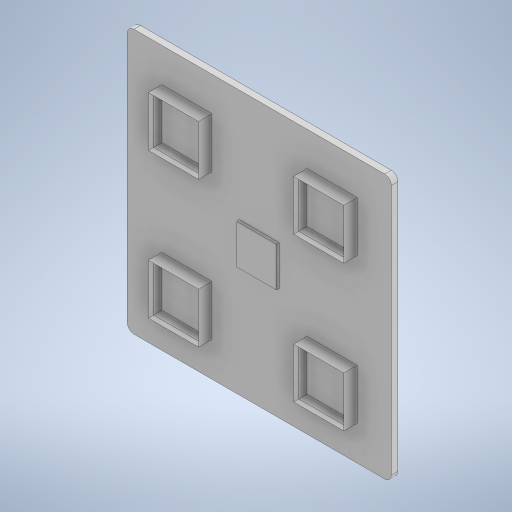
# Autodesk Inventor part: testovaci_podlozka
Saved by Autodesk Inventor 2023 (Build 270158000, 158)
## iProperties
Created: 2025-03-28
Part Number: testovaci_podlozka
Material: Všeobecné
Document SubType Name: Modeling
Designer: lisnik
Density: 1 g/cm^3
Appearance: Výchozí
Author: lisnik
Autodesk Inventor part; units mm, degrees
ref_plane "YZ Plane" through (0, 0, 0) normal (1, 0, 0) x (0, 1, 0)
ref_plane "XZ Plane" through (0, 0, 0) normal (0, 1, 0) x (-1, 0, 0)
ref_plane "XY Plane" through (0, 0, 0) normal (0, 0, 1) x (1, 0, 0)
sketch "Náčrt1" plane through (0, 0, 0) normal (0, 0, 1) x (1, 0, 0)
  line L0 (-140, 0) -> (140, 0) projected
  line L1 (0, -140) -> (0, 140) projected
  line L2 (-100, 100) -> (100, 100)
  line L3 (100, 100) -> (100, -100)
  line L4 (100, -100) -> (-100, -100)
  line L5 (-100, -100) -> (-100, 100)
  point P0 (0, 0)
  point P1 (0, 100)
  point P2 (100, 0)
  dimension "d0" = 200
  dimension "d1" = 200
  constraints: 8 end point, 2 midpoint, 2 parallel, 2 point on line, 1 horizontal, 1 perpendicular
  measures "d0" distance of L3.end L4.end
  measures "d1" distance of L2.end L3.end
extrude "Vysunutí1" add sketch "Náčrt1" along normal blind 5
fillet "Zaoblení1" radius 5 4 edges at (100, 100, 2.5) (-100, 100, 2.5) (-100, -100, 2.5) (100, -100, 2.5)
sketch "Náčrt2" plane through (0, 0, 5) normal (0, 0, 1) x (1, 0, 0)
  line L0 (-100, 95) -> (-100, -95) projected
  line L1 (-95, -100) -> (95, -100) projected
  arc A0 (95, -100) -> (100, -95) centre (95, -95) ccw projected
  line L2 (100, -95) -> (100, 95) projected
  arc A1 (100, 95) -> (95, 100) centre (95, 95) ccw projected
  line L3 (95, 100) -> (-95, 100) projected
  arc A2 (-95, 100) -> (-100, 95) centre (-95, 95) ccw projected
  line L4 (-100, 95) -> (-100, -95) projected
  arc A3 (-100, -95) -> (-95, -100) centre (-95, -95) ccw projected
  line L5 (-95, -100) -> (95, -100) projected
  line L6 (-141.4497, 0) -> (141.4497, 0) projected
  line L7 (0, -141.4497) -> (0, 141.4497) projected
  line L8 (-15, -15) -> (15, -15)
  line L9 (15, -15) -> (15, 15)
  line L10 (15, 15) -> (-15, 15)
  line L11 (-15, 15) -> (-15, -15)
  line L12 (-72, -72) -> (-38, -72)
  line L13 (-38, -72) -> (-38, -38)
  line L14 (-38, -38) -> (-72, -38)
  line L15 (-72, -38) -> (-72, -72)
  line L16 (-72, 38) -> (-38, 38)
  line L17 (-72, 72) -> (-72, 38)
  line L18 (-38, 72) -> (-72, 72)
  line L19 (-38, 38) -> (-38, 72)
  line L20 (38, -72) -> (72, -72)
  line L21 (38, -38) -> (38, -72)
  line L22 (72, -38) -> (38, -38)
  line L23 (72, -72) -> (72, -38)
  line L24 (38, 38) -> (72, 38)
  line L25 (38, 72) -> (38, 38)
  line L26 (72, 72) -> (38, 72)
  line L27 (72, 38) -> (72, 72)
  point P0 (0, 0)
  point P1 (-15, 0)
  point P2 (0, 15)
  dimension "d5" = 30
  dimension "d6" = 30
  dimension "d8" = 34
  dimension "d9" = 34
  dimension "d10" = 28
  dimension "d11" = 28
  dimension "d14" = 110
  dimension "d17" = 110
  constraints: 40 end point, 4 parallel, 3 horizontal, 2 midpoint, 2 perpendicular, 2 point on line, 1 vertical, 24 other
  measures "d5" distance of L8.end L9.end
  measures "d6" distance of L9.end L10.end
  measures "d8" distance of L13.start L13.end
  measures "d9" distance of L13.end L14.end
  measures "d10" distance between parallel lines of L5 L12
  measures "d11" distance between parallel lines of L0 L15
  measures "d14" distance of L15.end L16.start
  measures "d17" distance of L15.end L20.start
extrude "Vysunutí2" add sketch "Náčrt2" along normal blind 2 contours L11 L10 L7 L6 | L6 L7 L8 L11 | L7 L10 L9 L6 | L6 L9 L8 L7 | L15 L14 L13 L12 | L17 L18 L19 L16 | L21 L22 L23 L20 | L25 L26 L27 L24
sketch "Náčrt4" plane through (0, 0, 5) normal (0, 0, 1) x (1, 0, 0)
  line L0 (-38, 38) -> (-72, 38) projected
  line L1 (-72, 38) -> (-72, 72) projected
  line L2 (-72, 72) -> (-38, 72) projected
  line L3 (-38, 72) -> (-38, 38) projected
  line L4 (72, 38) -> (38, 38) projected
  line L5 (38, 38) -> (38, 72) projected
  line L6 (38, 72) -> (72, 72) projected
  line L7 (72, 72) -> (72, 38) projected
  line L8 (-15, 15) -> (15, 15) projected
  line L9 (15, 15) -> (15, -15) projected
  line L10 (15, -15) -> (-15, -15) projected
  line L11 (-15, -15) -> (-15, 15) projected
  line L12 (72, -72) -> (38, -72) projected
  line L13 (38, -72) -> (38, -38) projected
  line L14 (38, -38) -> (72, -38) projected
  line L15 (72, -38) -> (72, -72) projected
  line L16 (-38, -38) -> (-38, -72) projected
  line L17 (-38, -72) -> (-72, -72) projected
  line L18 (-72, -72) -> (-72, -38) projected
  line L19 (-72, -38) -> (-38, -38) projected
  arc A0 (95, -100) -> (100, -95) centre (95, -95) ccw projected
  line L20 (100, -95) -> (100, 95) projected
  arc A1 (100, 95) -> (95, 100) centre (95, 95) ccw projected
  line L21 (95, 100) -> (-95, 100) projected
  arc A2 (-95, 100) -> (-100, 95) centre (-95, 95) ccw projected
  line L22 (-100, 95) -> (-100, -95) projected
  arc A3 (-100, -95) -> (-95, -100) centre (-95, -95) ccw projected
  line L23 (-95, -100) -> (95, -100) projected
  line L24 (-38, -38) -> (-72, -38) projected
  line L25 (-72, -38) -> (-72, -72) projected
  line L26 (-72, -72) -> (-38, -72) projected
  line L27 (-38, -72) -> (-38, -38) projected
  line L28 (-15, 15) -> (-15, -15) projected
  line L29 (-15, -15) -> (15, -15) projected
  line L30 (15, -15) -> (15, 15) projected
  line L31 (15, 15) -> (-15, 15) projected
  line L32 (-38, 72) -> (-72, 72) projected
  line L33 (-38, 38) -> (-38, 72) projected
  line L34 (-38, 72) -> (-72, 72) projected
  line L35 (-72, 72) -> (-72, 38) projected
  line L36 (-72, 38) -> (-38, 38) projected
  line L37 (72, 38) -> (72, 72) projected
  line L38 (72, 72) -> (38, 72) projected
  line L39 (38, 72) -> (38, 38) projected
  line L40 (38, 38) -> (72, 38) projected
  line L41 (72, -72) -> (72, -38) projected
  line L42 (72, -38) -> (38, -38) projected
  line L43 (38, -38) -> (38, -72) projected
  line L44 (38, -72) -> (72, -72) projected
  line L45 (0, -141.4497) -> (0, 141.4497) projected
  line L46 (-141.4497, 0) -> (141.4497, 0) projected
  line L47 (-74, -74) -> (-36, -74)
  line L48 (-36, -74) -> (-36, -36)
  line L49 (-36, -36) -> (-74, -36)
  line L50 (-74, -36) -> (-74, -74)
  line L51 (-36, 36) -> (-36, 74)
  line L52 (-74, 36) -> (-36, 36)
  line L53 (-36, 74) -> (-74, 74)
  line L54 (-74, 74) -> (-74, 36)
  line L55 (74, -74) -> (74, -36)
  line L56 (36, -74) -> (74, -74)
  line L57 (74, -36) -> (36, -36)
  line L58 (36, -36) -> (36, -74)
  line L59 (74, 36) -> (74, 74)
  line L60 (36, 36) -> (74, 36)
  line L61 (74, 74) -> (36, 74)
  line L62 (36, 74) -> (36, 36)
  point P0 (0, 0)
  dimension "d22" = 38
  dimension "d23" = 38
  dimension "d24" = 2
  dimension "d25" = 2
  dimension "d28" = 110
  dimension "d31" = 110
  constraints: 32 end point, 2 horizontal, 2 parallel, 1 perpendicular, 1 vertical, 24 other
  measures "d22" distance of L47.end L48.end
  measures "d23" distance of L48.end L49.end
  measures "d24" distance between parallel lines of L48 L16
  measures "d25" distance between parallel lines of L49 L24
  measures "d28" distance of L47.end L51.start
  measures "d31" distance of L47.end L55.start
extrude "Vysunutí3" add sketch "Náčrt4" along normal blind 10 contours L50 L49 L48 L47 | L52 L54 L53 L51 | L56 L58 L57 L55 | L60 L62 L61 L59
chamfer "Zkosení1" distance 2 angle 45 16 edges at (-55, -72, 15) (-72, -55, 15) (-55, -38, 15) (-38, -55, 15) (-55, 38, 15) (-72, 55, 15) (-55, 72, 15) (-38, 55, 15) (38, -55, 15) (55, -38, 15) (55, -72, 15) (72, -55, 15) (55, 38, 15) (38, 55, 15) (55, 72, 15) (72, 55, 15)
